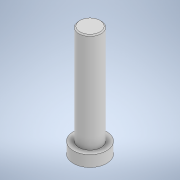
# Autodesk Inventor part: Trzpień
Saved by Autodesk Inventor 2021 (Build 250183000, 183)
## iProperties
Created: 2021-05-12
Part Number: Trzpień
Material: Ogólny
Document SubType Name: Modeling
Designer: DESKTOP-12
Density: 1 g/cm^3
Appearance: Domyślna
Author: DESKTOP-12
Autodesk Inventor part; units mm, degrees
ref_plane "YZ Plane" through (0, 0, 0) normal (1, 0, 0) x (0, 1, 0)
ref_plane "XZ Plane" through (0, 0, 0) normal (0, 1, 0) x (-1, 0, 0)
ref_plane "XY Plane" through (0, 0, 0) normal (0, 0, 1) x (1, 0, 0)
sketch "Szkic1" plane through (0, 0, 0) normal (0, 1, 0) x (-1, 0, 0)
  circle A0 centre (0, 0) radius 7.5
  dimension "d0" = 15
  constraints: 1 centre point, 1 coincident
  measures "d0" diameter of A0
extrude "Wyciągnięcie proste1" add sketch "Szkic1" along normal blind 5
sketch "Szkic2" plane through (0, 5, 0) normal (0, 1, 0) x (1, 0, 0)
  circle A0 centre (0, 0) radius 5
  dimension "d3" = 10
  constraints: 1 centre point, 1 coincident
  measures "d3" diameter of A0
extrude "Wyciągnięcie proste2" add sketch "Szkic2" along normal blind 45
chamfer "Faza1" distance 0.5 angle 45 1 edges at (-5, 50, 0)
sketch "Szkic3" plane through (0, 50, 0) normal (0, 1, 0) x (1, 0, 0)
  line L0 (-4.5, -5) -> (-5.5, -5)
  line L1 (-5.5, -5) -> (-5.5, 5)
  line L2 (-5.5, 5) -> (-4.5, 5)
  line L3 (-4.5, -5) -> (-4.5, 5)
  circle A0 centre (0, 0) radius 4.5 projected
  dimension "d10" = 1
  dimension "d11" = 10
  constraints: 8 end point, 2 perpendicular, 1 tangent, 1 vertical
  measures "d10" distance of L0.start L0.end
  measures "d11" distance of L0.end L1.end
extrude "Wyciągnięcie proste3" cut sketch "Szkic3" against normal blind 6 contours L0 L1 L2 L3
sketch "Szkic4" plane through (-4.5, 44, 2.1794) normal (-1, 0, 0) x (0, 0, 1)
  point P0 (-2.1794, -44)
  point P1 (-2.1794, 3)
hole "Otwór1" at (-4.5, 47, 0) direction (1, 0, 0) diameter 2.459 depth 6 tip angle 118 thread size "M3x0.5" class "6H" standard "ISO Metric profile"
